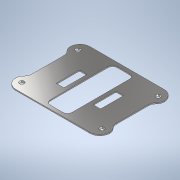
# Autodesk Inventor part: spacer
Saved by Autodesk Inventor 2022 (Build 260153000, 153)
## iProperties
Created: 2021-07-16
Part Number: spacer
Material: Stainless Steel
Document SubType Name: Modeling
Designer: Caleb
Density: 8 g/cm^3
Appearance: Semi-Polished
Author: Caleb
Autodesk Inventor part; units mm, degrees
ref_plane "YZ Plane" through (0, 0, 0) normal (1, 0, 0) x (0, 1, 0)
ref_plane "XZ Plane" through (0, 0, 0) normal (0, 1, 0) x (-1, 0, 0)
ref_plane "XY Plane" through (0, 0, 0) normal (0, 0, 1) x (1, 0, 0)
sketch "Sketch1" plane through (0, 0, 0) normal (0, 1, 0) x (-1, 0, 0)
  line L0 (-23.8125, 23.8125) -> (23.8125, 23.8125)
  line L1 (30.1625, 17.4625) -> (30.1625, -17.4625)
  line L2 (23.8125, -23.8125) -> (-23.8125, -23.8125)
  line L3 (-30.1625, -17.4625) -> (-30.1625, 17.4625)
  line L4 (-30.1625, 23.8125) -> (30.1625, -23.8125) construction
  line L5 (30.1625, 23.8125) -> (-30.1625, -23.8125) construction
  arc A0 (30.1625, 17.4625) -> (23.8125, 23.8125) centre (23.8125, 17.4625) ccw
  arc A1 (23.8125, -23.8125) -> (30.1625, -17.4625) centre (23.8125, -17.4625) ccw
  arc A2 (-30.1625, -17.4625) -> (-23.8125, -23.8125) centre (-23.8125, -17.4625) ccw
  arc A3 (-23.8125, 23.8125) -> (-30.1625, 17.4625) centre (-23.8125, 17.4625) ccw
  point P0 (0, 0)
  dimension "d0" = 47.625
  dimension "d1" = 60.325
  dimension "d2" = 6.35
  constraints: 12 end point, 8 point on circle, 8 point on line, 8 tangent, 4 centre point, 3 equal radius, 2 midpoint, 2 parallel, 1 horizontal, 1 perpendicular
  measures "d0" distance of L5.start L4.end
  measures "d1" distance of L4.end L5.end
  measures "d2" radius of A0
extrude "Extrusion1" add sketch "Sketch1" along normal blind 0.7
sketch "Sketch2" plane through (0, 0.7, 0) normal (0, 1, 0) x (1, 0, 0)
  point P0 (0, 0)
  point P1 (-25.75, 18.05)
  point P2 (25.75, 18.05)
  point P3 (-25.75, -18.05)
  point P4 (25.75, -18.05)
  dimension "d76" = 51.5
  dimension "d77" = 36.1
  dimension "d78" = 18.05
  dimension "d79" = 25.75
  constraints: 2 horizontal alignment, 2 vertical alignment
  measures "d76" distance of point (25.75, 18.05) point (-25.75, 18.05)
  measures "d77" distance of point (-25.75, -18.05) point (-25.75, 18.05)
  measures "d78" vertical distance of point (-25.75, 18.05) point (0, 0)
  measures "d79" horizontal distance of point (-25.75, 18.05) point (0, 0)
hole "Hole1" at (-25.75, 0.7, -18.05) at (25.75, 0.7, -18.05) at (-25.75, 0.7, 18.05) at (25.75, 0.7, 18.05) direction (0, -1, 0) diameter 1.778 end through all countersink diameter 3.023 countersink angle 82 clearance for "Flat Head Machine Screw (82)" size "#0" standard "Ansi Unified Screw Threads"
sketch "Sketch3" plane through (0, 0.7, 0) normal (0, 1, 0) x (1, 0, 0)
  line L0 (-9.7655, -7.5) -> (-13.7655, -7.5)
  line L1 (-14.2655, -7) -> (-14.2655, 7)
  line L2 (-13.7655, 7.5) -> (-9.7655, 7.5)
  line L3 (-9.2655, 7) -> (-9.2655, -7)
  line L4 (-9.2655, -7.5) -> (-14.2655, 7.5) construction
  line L5 (-14.2655, -7.5) -> (-9.2655, 7.5) construction
  line L6 (13.7655, -7.5) -> (9.7655, -7.5)
  line L7 (9.2655, -7) -> (9.2655, 7)
  line L8 (9.7655, 7.5) -> (13.7655, 7.5)
  line L9 (14.2655, 7) -> (14.2655, -7)
  line L10 (14.2655, -7.5) -> (9.2655, 7.5) construction
  line L11 (9.2655, -7.5) -> (14.2655, 7.5) construction
  arc A0 (-14.2655, -7) -> (-13.7655, -7.5) centre (-13.7655, -7) ccw
  arc A1 (-9.7655, -7.5) -> (-9.2655, -7) centre (-9.7655, -7) ccw
  arc A2 (-9.2655, 7) -> (-9.7655, 7.5) centre (-9.7655, 7) ccw
  arc A3 (-13.7655, 7.5) -> (-14.2655, 7) centre (-13.7655, 7) ccw
  arc A4 (9.2655, -7) -> (9.7655, -7.5) centre (9.7655, -7) ccw
  arc A5 (13.7655, -7.5) -> (14.2655, -7) centre (13.7655, -7) ccw
  arc A6 (14.2655, 7) -> (13.7655, 7.5) centre (13.7655, 7) ccw
  arc A7 (9.7655, 7.5) -> (9.2655, 7) centre (9.7655, 7) ccw
  point P0 (0, 0)
  point P1 (-11.7655, 0)
  point P2 (11.7655, 0)
  point P3 (-11.7655, 0)
  point P4 (11.7655, 0)
  point P5 (-11.7655, 0)
  dimension "d18" = 15
  dimension "d21" = 5
  dimension "d72" = 23.531
  dimension "d73" = 11.7655
  dimension "d85" = 0.5
  dimension "d86" = 0.5
  constraints: 24 end point, 16 point on circle, 16 point on line, 16 tangent, 8 centre point, 7 midpoint, 6 equal radius, 4 parallel, 2 equal length, 2 horizontal, 2 horizontal alignment, 2 perpendicular, 1 coincident
  measures "d18" distance of L5.start L4.end
  measures "d21" distance of L4.start L5.start
  measures "d72" distance of point (11.765, 0) point (-11.765, 0)
  measures "d73" distance of point (-11.765, 0) point (0, 0)
  measures "d85" radius of A0
  measures "d86" radius of A1
extrude "Extrusion2" cut sketch "Sketch3" against normal through all
sketch "Sketch5" plane through (0, 0.7, 0) normal (0, 1, 0) x (1, 0, 0)
  line L0 (-30.1625, 17.4625) -> (-30.1625, -17.4625) projected
  line L1 (30.1625, -17.4625) -> (30.1625, 17.4625) projected
  arc A0 (-23.8125, 23.8125) -> (-30.1625, 17.4625) centre (-23.8125, 17.4625) ccw projected
  arc A1 (-30.1625, -17.4625) -> (-23.8125, -23.8125) centre (-23.8125, -17.4625) ccw projected
  arc A2 (-28.6746, -13.8704) -> (-30.1625, -17.4625) centre (-25.0825, -17.4625) ccw
  line L2 (-30.1625, -17.4625) -> (-25.0825, -17.4625) construction
  line L3 (-28.6746, -13.8704) -> (-25.0825, -17.4625) construction
  arc A3 (-28.6746, -13.8704) -> (-27.1867, -10.2783) centre (-32.2667, -10.2783) ccw
  line L4 (-28.6746, -13.8704) -> (-32.2667, -10.2783) construction
  line L5 (-27.1867, -10.2783) -> (-32.2667, -10.2783) construction
  arc A4 (-30.1625, 17.4625) -> (-28.6746, 13.8704) centre (-25.0825, 17.4625) ccw
  line L6 (-30.1625, 17.4625) -> (-25.0825, 17.4625) construction
  line L7 (-28.6746, 13.8704) -> (-25.0825, 17.4625) construction
  arc A5 (-27.1867, 10.2783) -> (-28.6746, 13.8704) centre (-32.2667, 10.2783) ccw
  line L8 (-28.6746, 13.8704) -> (-32.2667, 10.2783) construction
  line L9 (-27.1867, 10.2783) -> (-32.2667, 10.2783) construction
  line L10 (-27.1867, 10.2783) -> (-27.1867, -10.2783)
  arc A6 (30.1625, 17.4625) -> (23.8125, 23.8125) centre (23.8125, 17.4625) ccw projected
  arc A7 (23.8125, -23.8125) -> (30.1625, -17.4625) centre (23.8125, -17.4625) ccw projected
  arc A8 (28.6746, 13.8704) -> (30.1625, 17.4625) centre (25.0825, 17.4625) ccw
  line L11 (30.1625, 17.4625) -> (25.0825, 17.4625) construction
  line L12 (28.6746, 13.8704) -> (25.0825, 17.4625) construction
  arc A9 (28.6746, 13.8704) -> (27.1867, 10.2783) centre (32.2667, 10.2783) ccw
  line L13 (28.6746, 13.8704) -> (32.2667, 10.2783) construction
  line L14 (27.1867, 10.2783) -> (32.2667, 10.2783) construction
  arc A10 (30.1625, -17.4625) -> (28.6746, -13.8704) centre (25.0825, -17.4625) ccw
  line L15 (30.1625, -17.4625) -> (25.0825, -17.4625) construction
  line L16 (28.6746, -13.8704) -> (25.0825, -17.4625) construction
  arc A11 (27.1867, -10.2783) -> (28.6746, -13.8704) centre (32.2667, -10.2783) ccw
  line L17 (28.6746, -13.8704) -> (32.2667, -10.2783) construction
  line L18 (27.1867, -10.2783) -> (32.2667, -10.2783) construction
  line L19 (27.1867, -10.2783) -> (27.1867, 10.2783)
  point P0 (0, 0)
  dimension "d41" = 5.08
  dimension "d42" = 45
  dimension "d43" = 5.08
  dimension "d44" = 45
  dimension "d45" = 5.08
  dimension "d46" = 45
  dimension "d47" = 5.08
  dimension "d48" = 45
  dimension "d51" = 5.08
  dimension "d52" = 45
  dimension "d53" = 5.08
  dimension "d54" = 45
  dimension "d57" = 5.08
  dimension "d58" = 45
  dimension "d59" = 5.08
  dimension "d60" = 45
  constraints: 36 end point, 16 point on circle, 8 centre point, 8 tangent
  measures "d41" radius of A2
  measures "d42" angle of L3 L2
  measures "d43" radius of A3
  measures "d44" angle of L4 L5
  measures "d45" radius of A4
  measures "d46" angle of L6 L7
  measures "d47" radius of A5
  measures "d48" angle of L9 L8
  measures "d51" radius of A8
  measures "d52" angle of L12 L11
  measures "d53" radius of A9
  measures "d54" angle of L13 L14
  measures "d57" radius of A10
  measures "d58" angle of L15 L16
  measures "d59" radius of A11
  measures "d60" angle of L18 L17
extrude "Extrusion3" cut sketch "Sketch5" against normal through all
sketch "Sketch7" plane through (0, 0.7, 0) normal (0, 1, 0) x (1, 0, 0)
  line L0 (4, 21.5) -> (-4, 21.5)
  line L1 (-7, 18.5) -> (-7, -18.5)
  line L2 (-4, -21.5) -> (4, -21.5)
  line L3 (7, -18.5) -> (7, 18.5)
  line L4 (7, 21.5) -> (-7, -21.5) construction
  line L5 (-7, 21.5) -> (7, -21.5) construction
  arc A0 (-7, -18.5) -> (-4, -21.5) centre (-4, -18.5) ccw
  arc A1 (4, -21.5) -> (7, -18.5) centre (4, -18.5) ccw
  arc A2 (7, 18.5) -> (4, 21.5) centre (4, 18.5) ccw
  arc A3 (-4, 21.5) -> (-7, 18.5) centre (-4, 18.5) ccw
  point P0 (0, 0)
  dimension "d80" = 14
  dimension "d81" = 43
  dimension "d82" = 3
  constraints: 12 end point, 8 point on circle, 8 point on line, 8 tangent, 4 centre point, 3 equal radius, 2 midpoint, 2 parallel, 1 horizontal, 1 perpendicular
  measures "d80" distance of L5.end L4.end
  measures "d81" distance of L4.end L5.start
  measures "d82" radius of A0
extrude "Extrusion4" cut sketch "Sketch7" against normal through all
body "Solid1"
